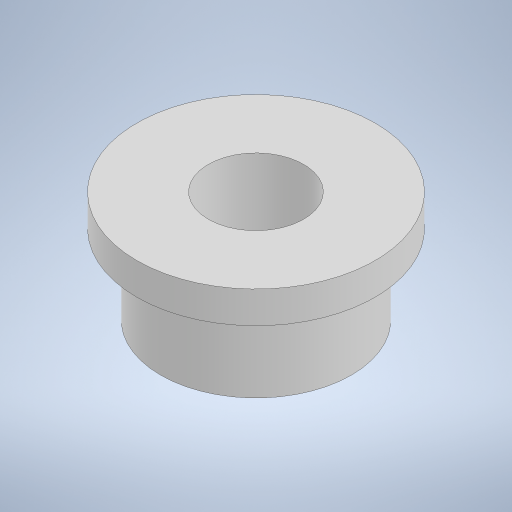
# Autodesk Inventor part: adder
Saved by Autodesk Inventor 2023 (Build 270158000, 158)
## iProperties
Created: 2024-06-09
Part Number: adder
Material: 常规
Document SubType Name: Modeling
Designer: Nitrene.P.L
Density: 1 g/cm^3
Appearance: 默认
Author: Nitrene.P.L
Autodesk Inventor part; units mm, degrees
ref_plane "YZ Plane" through (0, 0, 0) normal (1, 0, 0) x (0, 1, 0)
ref_plane "XZ Plane" through (0, 0, 0) normal (0, 1, 0) x (-1, 0, 0)
ref_plane "XY Plane" through (0, 0, 0) normal (0, 0, 1) x (1, 0, 0)
sketch "草图2" plane through (0, 0, 0) normal (1, 0, 0) x (0, 1, 0)
  line L0 (-3.5, 0) -> (3.5, 0)
  line L1 (3.5, 0) -> (3.5, 3)
  line L2 (3.5, 3) -> (-3.5, 3)
  line L3 (-3.5, 3) -> (-3.5, 0)
  line L4 (0, 1.8375) -> (0, -3)
  line L5 (-2.3352, 0) -> (1.7062, 0)
  line L6 (3.5, 3) -> (-3.5, 3)
  line L7 (-3.5, 3) -> (-3.5, 6)
  line L8 (-3.5, 6) -> (3.5, 6)
  line L9 (3.5, 6) -> (3.5, 3)
  line L10 (3.5, 6) -> (1.5, 6)
  line L11 (1.5, 6) -> (1.5, 7.5)
  line L12 (1.5, 7.5) -> (3.5, 7.5)
  line L13 (3.5, 7.5) -> (3.5, 6)
  point P0 (0, 0)
  dimension "d0" = 7
  dimension "d1" = 3
  dimension "d2" = 3
  dimension "d3" = 2
  dimension "d4" = 1.5
  constraints: 28 end point, 6 horizontal, 6 parallel, 3 perpendicular, 2 vertical, 1 collinear, 1 other
  measures "d0" distance of L1.end L2.end
  measures "d1" distance of L0.end L1.end
  measures "d2" distance of L6.end L7.end
  measures "d3" distance of L11.end L12.end
  measures "d4" distance of L10.end L11.end
revolve "旋转1" add sketch "草图2" angle 360 about axis through (0, -3.5, 0) along (0, 1, 0) contours L7 L8 L9 L2 | L8 L11 L12 L13
